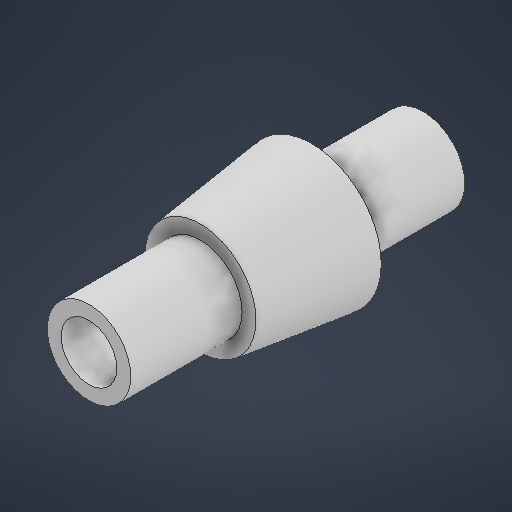
# Autodesk Inventor part: Tipo2
Saved by Autodesk Inventor 2026 (Build 300175050, 175E)
## iProperties
Created: 2026-04-09
Part Number: Tipo2
Material: Generic
Document SubType Name: Modeling
Designer: Administrator
Density: 1 g/cm^3
Appearance: Default
Author: Administrator
Autodesk Inventor part; units mm, degrees
ref_plane "YZ Plane" through (0, 0, 0) normal (1, 0, 0) x (0, 1, 0)
ref_plane "XZ Plane" through (0, 0, 0) normal (0, 1, 0) x (-1, 0, 0)
ref_plane "XY Plane" through (0, 0, 0) normal (0, 0, 1) x (1, 0, 0)
sketch "Sketch1" plane through (0, 0, 0) normal (0, 1, 0) x (-1, 0, 0)
  line L0 (0, 0) -> (0, -60)
  line L1 (0, -60) -> (7.5, -60)
  line L2 (7.5, -60) -> (7.5, -40)
  line L3 (7.5, -40) -> (12.5, -40)
  line L4 (10, -20) -> (7.5, -20)
  line L5 (7.5, -20) -> (7.5, 0)
  line L6 (7.5, 0) -> (0, 0)
  line L7 (10, -20) -> (12.5, -40)
  dimension "d1" = 60
  dimension "d2" = 15
  dimension "d3" = 20
  dimension "d4" = 25
  dimension "d5" = 15
  dimension "d6" = 40
  dimension "d7" = 20
  constraints: 16 end point, 5 perpendicular, 1 parallel, 1 vertical
  measures "d1" distance between parallel lines of L1 L6
  measures "d2" diameter of L5 L0
  measures "d3" vertical distance of L4.start L0
  measures "d4" diameter of L3.end L0
  measures "d5" diameter of L2 L0
  measures "d6" distance between parallel lines of L1 L4
  measures "d7" distance between parallel lines of L1 L3
revolve "Revolution1" add sketch "Sketch1" angle 360 mid plane about axis through (0, 0, 0) along (0, 0, -1)
sketch "Sketch2" plane through (0, 0, 0) normal (0, 0, 1) x (1, 0, 0)
  circle A0 centre (0, 0) radius 5
  dimension "d9" = 10
  constraints: 1 centre point, 1 coincident
  measures "d9" diameter of A0
extrude "Extrusion1" cut sketch "Sketch2" against normal blind 60
body "Solid1"
